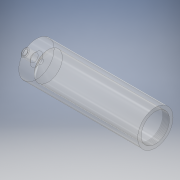
# Autodesk Inventor part: PayloadGermination_Syringe
Saved by Autodesk Inventor 2018 (Build 220112000, 112)
## iProperties
Created: 2018-07-29
Part Number: PayloadGermination_Syringe
Material: Polycarbonate, Clear
Document SubType Name: Modeling
Designer: Bradley
Density: 1.2 g/cm^3
Appearance: Polycarbonate - Clear
Author: Bradley
Autodesk Inventor part; units mm, degrees
ref_plane "YZ Plane" through (0, 0, 0) normal (1, 0, 0) x (0, 1, 0)
ref_plane "XZ Plane" through (0, 0, 0) normal (0, 1, 0) x (-1, 0, 0)
ref_plane "XY Plane" through (0, 0, 0) normal (0, 0, 1) x (1, 0, 0)
sketch "Sketch1" plane through (0, 0, 0) normal (0, 1, 0) x (-1, 0, 0)
  line L0 (22.7522, 7.5) -> (-27.7522, 7.5)
  line L1 (-27.7522, 7.5) -> (-27.7522, 6)
  line L2 (-27.7522, 6) -> (17.7478, 6)
  line L3 (17.7478, 6) -> (20.7522, 1)
  line L4 (20.7522, 1) -> (27.7522, 1)
  line L5 (27.7522, 1) -> (27.7522, 1.75)
  line L6 (27.7522, 1.75) -> (22.7522, 1.75)
  line L7 (22.7522, 1.75) -> (22.7522, 7.5)
  line L8 (27.7522, 0) -> (-27.7522, 0)
  point P0 (0, 0)
  point P1 (0, 0)
  dimension "d0" = 2
  dimension "d1" = 3.5
  dimension "d2" = 5
  dimension "d3" = 59
  dimension "d5" = 1.5
  dimension "d6" = 2
  dimension "d13" = 12
  dimension "d14" = 45.5
  constraints: 18 end point, 3 perpendicular, 2 horizontal, 2 point on line, 1 coincident, 1 midpoint, 1 parallel, 1 vertical
  measures "d0" diameter of L4 L8
  measures "d1" diameter of L6 L8
  measures "d2" distance of L5.end L6.end
  measures "d3" angle of L8 L3
  measures "d5" distance between parallel lines of L2 L0
  measures "d6" distance from line of L7 L3.end
  measures "d13" diameter of L2 L8
  measures "d14" distance of L1.end L2.end
revolve "Revolution1" add sketch "Sketch1" angle 360 about axis through (-27.7522, 0, 0) along (1, 0, 0)
fillet "Fillet1" radius 1 1 edges at (-22.7522, 0, -1.75)
fillet "Fillet1" radius 0.25 2 edges at (-27.7522, 0, -1.75) (-27.7522, 0, -1)
thread "Thread1" size "M12x0.5" class "6H" standard "ANSI Metric M Profile" length 3
body "Solid1"
